Autodesk Fusion 360 part; units mm, degrees
note: some values were not read from the file. Chosen so that the rebuilt part matches the saved one: which bodies a step acts on; a direction. Set by a fixed rule: which sketch regions a step uses.
(part 2 of 5)
sketch "ToF block FL sketch" plane through (0, 0, 0) normal (0, 0, 1) x (1, 0, 0) in component "Upper frame"
  line L0 (88.4256, 25.8962) -> (99.9126, 31.2979)
  line L1 (99.9126, 31.2979) -> (89.9042, 53.4861)
  line L2 (89.9042, 53.4861) -> (78.1222, 47.992)
  line L3 (78.1222, 47.992) -> (88.4256, 25.8962)
extrude "ToF block FL" add sketch "ToF block FL sketch" along normal blind 30 from surface at 87 bodies 44 in component "Upper frame"
sketch "ToF block FR sketch" plane through (0, 0, 0) normal (0, 0, 1) x (1, 0, 0) in component "Upper frame"
  line L0 (78.1222, -47.992) -> (89.9042, -53.4861)
  line L1 (89.9042, -53.4861) -> (99.9126, -31.2979)
  line L2 (99.9126, -31.2979) -> (88.4256, -25.8962)
  line L3 (88.4256, -25.8962) -> (78.1222, -47.992)
extrude "ToF block FR" add sketch "ToF block FR sketch" along normal blind 30 from surface at 87 bodies 44 in component "Upper frame"
sketch "ToF block SFL sketch" plane through (0, 0, 0) normal (0, 0, 1) x (1, 0, 0) in component "Upper frame"
  line L0 (80.69, 53.1) -> (80.69, 66.1)
  line L1 (80.69, 66.1) -> (56.31, 66.1)
  line L2 (56.31, 66.1) -> (56.31, 53.1)
  line L3 (56.31, 53.1) -> (80.69, 53.1)
extrude "ToF block SFL" add sketch "ToF block SFL sketch" along normal blind 30 from surface at 87 bodies 44 in component "Upper frame"
sketch "ToF block SFR sketch" plane through (0, 0, 0) normal (0, 0, 1) x (1, 0, 0) in component "Upper frame"
  line L0 (56.31, -53.1) -> (56.31, -66.1)
  line L1 (56.31, -66.1) -> (80.69, -66.1)
  line L2 (80.69, -66.1) -> (80.69, -53.1)
  line L3 (80.69, -53.1) -> (56.31, -53.1)
extrude "ToF block SFR" add sketch "ToF block SFR sketch" along normal blind 30 from surface at 87 bodies 44 in component "Upper frame"
sketch "ToF block SRL sketch" plane through (0, 0, 0) normal (0, 0, 1) x (1, 0, 0) in component "Upper frame"
  line L0 (-56.31, 53.1) -> (-56.31, 66.1)
  line L1 (-56.31, 66.1) -> (-80.69, 66.1)
  line L2 (-80.69, 66.1) -> (-80.69, 53.1)
  line L3 (-80.69, 53.1) -> (-56.31, 53.1)
extrude "ToF block SRL" add sketch "ToF block SRL sketch" along normal blind 30 from surface at 87 bodies 44 in component "Upper frame"
sketch "ToF block SRR sketch" plane through (0, 0, 0) normal (0, 0, 1) x (1, 0, 0) in component "Upper frame"
  line L0 (-80.69, -53.1) -> (-80.69, -66.1)
  line L1 (-80.69, -66.1) -> (-56.31, -66.1)
  line L2 (-56.31, -66.1) -> (-56.31, -53.1)
  line L3 (-56.31, -53.1) -> (-80.69, -53.1)
extrude "ToF block SRR" add sketch "ToF block SRR sketch" along normal blind 30 from surface at 87 bodies 44 in component "Upper frame"
sketch "ToF block RL sketch" plane through (0, 0, 0) normal (0, 0, 1) x (1, 0, 0) in component "Upper frame"
  line L0 (-77.1, 48.19) -> (-90.1, 48.19)
  line L1 (-90.1, 48.19) -> (-90.1, 23.81)
  line L2 (-90.1, 23.81) -> (-77.1, 23.81)
  line L3 (-77.1, 23.81) -> (-77.1, 48.19)
extrude "ToF block RL" add sketch "ToF block RL sketch" along normal blind 30 from surface at 87 bodies 44 in component "Upper frame"
sketch "ToF block RR sketch" plane through (0, 0, 0) normal (0, 0, 1) x (1, 0, 0) in component "Upper frame"
  line L0 (-77.1, -23.81) -> (-90.1, -23.81)
  line L1 (-90.1, -23.81) -> (-90.1, -48.19)
  line L2 (-90.1, -48.19) -> (-77.1, -48.19)
  line L3 (-77.1, -48.19) -> (-77.1, -23.81)
extrude "ToF block RR" add sketch "ToF block RR sketch" along normal blind 30 from surface at 87 bodies 44 in component "Upper frame"
sketch "Seat rebate 0 sketch" plane through (0, 0, 0) normal (0, 0, 1) x (1, 0, 0) in component "Upper frame"
  line L0 (31.5, 8) -> (39.5, 8)
  line L1 (39.5, 8) -> (39.5, 13)
  line L2 (39.5, 13) -> (31.5, 13)
  line L3 (31.5, 13) -> (31.5, 8)
extrude "Seat rebate 0" cut sketch "Seat rebate 0 sketch" along normal blind 2.5 from surface at 88.5 bodies 44 in component "Upper frame"
sketch "Seat rebate 1 sketch" plane through (0, 0, 0) normal (0, 0, 1) x (1, 0, 0) in component "Upper frame"
  line L0 (31.5, -13) -> (39.5, -13)
  line L1 (39.5, -13) -> (39.5, -8)
  line L2 (39.5, -8) -> (31.5, -8)
  line L3 (31.5, -8) -> (31.5, -13)
extrude "Seat rebate 1" cut sketch "Seat rebate 1 sketch" along normal blind 2.5 from surface at 88.5 bodies 44 in component "Upper frame"
sketch "Seat rebate 2 sketch" plane through (0, 0, 0) normal (0, 0, 1) x (1, 0, 0) in component "Upper frame"
  line L0 (-75.5, -5.5) -> (-71.5, -5.5)
  line L1 (-71.5, -5.5) -> (-71.5, 5.5)
  line L2 (-71.5, 5.5) -> (-75.5, 5.5)
  line L3 (-75.5, 5.5) -> (-75.5, -5.5)
extrude "Seat rebate 2" cut sketch "Seat rebate 2 sketch" along normal blind 2.5 from surface at 88.5 bodies 44 in component "Upper frame"
sketch "Screw hole +12 sketch" plane through (0, 0, 0) normal (0, 0, 1) x (1, 0, 0) in component "Upper frame"
  circle A0 centre (95.3694, 20.2714) radius 1.65
extrude "Screw hole +12" cut sketch "Screw hole +12 sketch" along normal blind 32 from surface at 86 bodies 44 in component "Upper frame"
sketch "Screw counterbore +12 sketch" plane through (0, 0, 0) normal (0, 0, 1) x (1, 0, 0) in component "Upper frame"
  circle A0 centre (95.3694, 20.2714) radius 3
extrude "Screw counterbore +12" cut sketch "Screw counterbore +12 sketch" along normal blind 4 from surface at 114 bodies 44 in component "Upper frame"
sketch "Screw hole +60 sketch" plane through (0, 0, 0) normal (0, 0, 1) x (1, 0, 0) in component "Upper frame"
  circle A0 centre (48.75, 84.4375) radius 1.65
extrude "Screw hole +60" cut sketch "Screw hole +60 sketch" along normal blind 32 from surface at 86 bodies 44 in component "Upper frame"
sketch "Screw counterbore +60 sketch" plane through (0, 0, 0) normal (0, 0, 1) x (1, 0, 0) in component "Upper frame"
  circle A0 centre (48.75, 84.4375) radius 3
extrude "Screw counterbore +60" cut sketch "Screw counterbore +60 sketch" along normal blind 4 from surface at 114 bodies 44 in component "Upper frame"
sketch "Screw hole +118 sketch" plane through (0, 0, 0) normal (0, 0, 1) x (1, 0, 0) in component "Upper frame"
  circle A0 centre (-45.7735, 86.0874) radius 1.65
extrude "Screw hole +118" cut sketch "Screw hole +118 sketch" along normal blind 32 from surface at 86 bodies 44 in component "Upper frame"
sketch "Screw counterbore +118 sketch" plane through (0, 0, 0) normal (0, 0, 1) x (1, 0, 0) in component "Upper frame"
  circle A0 centre (-45.7735, 86.0874) radius 3
extrude "Screw counterbore +118" cut sketch "Screw counterbore +118 sketch" along normal blind 4 from surface at 114 bodies 44 in component "Upper frame"
sketch "Screw hole -12 sketch" plane through (0, 0, 0) normal (0, 0, 1) x (1, 0, 0) in component "Upper frame"
  circle A0 centre (95.3694, -20.2714) radius 1.65
extrude "Screw hole -12" cut sketch "Screw hole -12 sketch" along normal blind 32 from surface at 86 bodies 44 in component "Upper frame"
sketch "Screw counterbore -12 sketch" plane through (0, 0, 0) normal (0, 0, 1) x (1, 0, 0) in component "Upper frame"
  circle A0 centre (95.3694, -20.2714) radius 3
extrude "Screw counterbore -12" cut sketch "Screw counterbore -12 sketch" along normal blind 4 from surface at 114 bodies 44 in component "Upper frame"
sketch "Screw hole -60 sketch" plane through (0, 0, 0) normal (0, 0, 1) x (1, 0, 0) in component "Upper frame"
  circle A0 centre (48.75, -84.4375) radius 1.65
extrude "Screw hole -60" cut sketch "Screw hole -60 sketch" along normal blind 32 from surface at 86 bodies 44 in component "Upper frame"
sketch "Screw counterbore -60 sketch" plane through (0, 0, 0) normal (0, 0, 1) x (1, 0, 0) in component "Upper frame"
  circle A0 centre (48.75, -84.4375) radius 3
extrude "Screw counterbore -60" cut sketch "Screw counterbore -60 sketch" along normal blind 4 from surface at 114 bodies 44 in component "Upper frame"
sketch "Screw hole -118 sketch" plane through (0, 0, 0) normal (0, 0, 1) x (1, 0, 0) in component "Upper frame"
  circle A0 centre (-45.7735, -86.0874) radius 1.65
extrude "Screw hole -118" cut sketch "Screw hole -118 sketch" along normal blind 32 from surface at 86 bodies 44 in component "Upper frame"
sketch "Screw counterbore -118 sketch" plane through (0, 0, 0) normal (0, 0, 1) x (1, 0, 0) in component "Upper frame"
  circle A0 centre (-45.7735, -86.0874) radius 3
extrude "Screw counterbore -118" cut sketch "Screw counterbore -118 sketch" along normal blind 4 from surface at 114 bodies 44 in component "Upper frame"
sketch "Hook rebate +71 sketch" plane through (0, 0, 0) normal (0, 0, 1) x (1, 0, 0) in component "Upper frame"
  arc A0 (44.7975, 96.0686) -> (23.8448, 103.2832) centre (0, 0) ccw
  line L0 (23.8448, 103.2832) -> (23.2599, 100.7499)
  arc A1 (43.6987, 93.7122) -> (23.2599, 100.7499) centre (0, 0) ccw
  line L1 (43.6987, 93.7122) -> (44.7975, 96.0686)
extrude "Hook rebate +71" cut sketch "Hook rebate +71 sketch" along normal blind 9 from surface at 109 bodies 44 in component "Upper frame"
sketch "Hook groove +71 sketch" plane through (0, 0, 0) normal (0, 0, 1) x (1, 0, 0) in component "Upper frame"
  arc A0 (41.2705, 94.9157) -> (25.9143, 100.2033) centre (0, 0) ccw
  line L0 (25.9143, 100.2033) -> (25.6389, 99.1383)
  arc A1 (40.8319, 93.907) -> (25.6389, 99.1383) centre (0, 0) ccw
  line L1 (40.8319, 93.907) -> (41.2705, 94.9157)
extrude "Hook groove +71" cut sketch "Hook groove +71 sketch" along normal blind 3 from surface at 110.5 bodies 44 in component "Upper frame"
sketch "Hook rebate +114 sketch" plane through (0, 0, 0) normal (0, 0, 1) x (1, 0, 0) in component "Upper frame"
  arc A0 (-32.7558, 100.812) -> (-53, 91.7987) centre (0, 0) ccw
  line L0 (-53, 91.7987) -> (-51.7, 89.547)
  arc A1 (-31.9524, 98.3392) -> (-51.7, 89.547) centre (0, 0) ccw
  line L1 (-31.9524, 98.3392) -> (-32.7558, 100.812)
extrude "Hook rebate +114" cut sketch "Hook rebate +114 sketch" along normal blind 9 from surface at 109 bodies 44 in component "Upper frame"
sketch "Hook groove +114 sketch" plane through (0, 0, 0) normal (0, 0, 1) x (1, 0, 0) in component "Upper frame"
  arc A0 (-34.549, 97.5634) -> (-49.3859, 90.9576) centre (0, 0) ccw
  line L0 (-49.3859, 90.9576) -> (-48.8611, 89.9909)
  arc A1 (-34.1818, 96.5265) -> (-48.8611, 89.9909) centre (0, 0) ccw
  line L1 (-34.1818, 96.5265) -> (-34.549, 97.5634)
extrude "Hook groove +114" cut sketch "Hook groove +114 sketch" along normal blind 3 from surface at 110.5 bodies 44 in component "Upper frame"
sketch "Hook rebate -71 sketch" plane through (0, 0, 0) normal (0, 0, 1) x (1, 0, 0) in component "Upper frame"
  arc A0 (23.8448, -103.2832) -> (44.7975, -96.0686) centre (0, 0) ccw
  line L0 (44.7975, -96.0686) -> (43.6987, -93.7122)
  arc A1 (23.2599, -100.7499) -> (43.6987, -93.7122) centre (0, 0) ccw
  line L1 (23.2599, -100.7499) -> (23.8448, -103.2832)
extrude "Hook rebate -71" cut sketch "Hook rebate -71 sketch" along normal blind 9 from surface at 109 bodies 44 in component "Upper frame"
sketch "Hook groove -71 sketch" plane through (0, 0, 0) normal (0, 0, 1) x (1, 0, 0) in component "Upper frame"
  arc A0 (25.9143, -100.2033) -> (41.2705, -94.9157) centre (0, 0) ccw
  line L0 (41.2705, -94.9157) -> (40.8319, -93.907)
  arc A1 (25.6389, -99.1383) -> (40.8319, -93.907) centre (0, 0) ccw
  line L1 (25.6389, -99.1383) -> (25.9143, -100.2033)
extrude "Hook groove -71" cut sketch "Hook groove -71 sketch" along normal blind 3 from surface at 110.5 bodies 44 in component "Upper frame"
sketch "Hook rebate -114 sketch" plane through (0, 0, 0) normal (0, 0, 1) x (1, 0, 0) in component "Upper frame"
  arc A0 (-53, -91.7987) -> (-32.7558, -100.812) centre (0, 0) ccw
  line L0 (-32.7558, -100.812) -> (-31.9524, -98.3392)
  arc A1 (-51.7, -89.547) -> (-31.9524, -98.3392) centre (0, 0) ccw
  line L1 (-51.7, -89.547) -> (-53, -91.7987)
extrude "Hook rebate -114" cut sketch "Hook rebate -114 sketch" along normal blind 9 from surface at 109 bodies 44 in component "Upper frame"
sketch "Hook groove -114 sketch" plane through (0, 0, 0) normal (0, 0, 1) x (1, 0, 0) in component "Upper frame"
  arc A0 (-49.3859, -90.9576) -> (-34.549, -97.5634) centre (0, 0) ccw
  line L0 (-34.549, -97.5634) -> (-34.1818, -96.5265)
  arc A1 (-48.8611, -89.9909) -> (-34.1818, -96.5265) centre (0, 0) ccw
  line L1 (-48.8611, -89.9909) -> (-49.3859, -90.9576)
extrude "Hook groove -114" cut sketch "Hook groove -114 sketch" along normal blind 3 from surface at 110.5 bodies 44 in component "Upper frame"
sketch "ToF pocket F sketch" plane through (0, 0, 0) normal (0, 0, 1) x (1, 0, 0) in component "Upper frame"
  line L0 (91.1, -9.69) -> (98.6, -9.69)
  line L1 (98.6, -9.69) -> (98.6, 9.69)
  line L2 (98.6, 9.69) -> (91.1, 9.69)
  line L3 (91.1, 9.69) -> (91.1, -9.69)
extrude "ToF pocket F" cut sketch "ToF pocket F sketch" along normal blind 28 from surface at 90 bodies 44 in component "Upper frame"
sketch "ToF plug shaft F sketch" plane through (0, 0, 0) normal (0, 0, 1) x (1, 0, 0) in component "Upper frame"
  line L0 (94.5, -3.8) -> (99, -3.8)
  line L1 (99, -3.8) -> (99, 3.8)
  line L2 (99, 3.8) -> (94.5, 3.8)
  line L3 (94.5, 3.8) -> (94.5, -3.8)
extrude "ToF plug shaft F" cut sketch "ToF plug shaft F sketch" along normal blind 4.5 from surface at 86 bodies 44 in component "Upper frame"
sketch "ToF tunnel F sketch" plane through (0, 0, 0) normal (0, 0, 1) x (1, 0, 0) in component "Upper frame"
  line L0 (98.1, -9) -> (135, -9)
  line L1 (135, -9) -> (135, 9)
  line L2 (135, 9) -> (98.1, 9)
  line L3 (98.1, 9) -> (98.1, -9)
extrude "ToF tunnel F" cut sketch "ToF tunnel F sketch" along normal blind 18 from surface at 93.8 bodies 44 in component "Upper frame"
sketch "ToF posts F sketch" plane through (0, 0, 0) normal (0, 0, 1) x (1, 0, 0) in component "Upper frame"
  line L0 (95, 3.75) -> (99.2, 3.75)
  line L1 (99.2, 3.75) -> (99.2, 8.95)
  line L2 (99.2, 8.95) -> (95, 8.95)
  line L3 (95, 8.95) -> (95, 3.75)
  line L4 (95, -8.95) -> (99.2, -8.95)
  line L5 (99.2, -8.95) -> (99.2, -3.75)
  line L6 (99.2, -3.75) -> (95, -3.75)
  line L7 (95, -3.75) -> (95, -8.95)
extrude "ToF posts F" add sketch "ToF posts F sketch" along normal blind 5.2 from surface at 110.36 bodies 44 in component "Upper frame"
sketch "ToF pilots F sketch" plane through (0, 0, 0) normal (0, 0, 1) x (1, 0, 0) in component "Upper frame"
  line L0 (94.5, 5.25) -> (99.5, 5.25)
  line L1 (99.5, 5.25) -> (99.5, 7.45)
  line L2 (99.5, 7.45) -> (94.5, 7.45)
  line L3 (94.5, 7.45) -> (94.5, 5.25)
  line L4 (94.5, -7.45) -> (99.5, -7.45)
  line L5 (99.5, -7.45) -> (99.5, -5.25)
  line L6 (99.5, -5.25) -> (94.5, -5.25)
  line L7 (94.5, -5.25) -> (94.5, -7.45)
extrude "ToF pilots F" cut sketch "ToF pilots F sketch" along normal blind 2.2 from surface at 111.86 bodies 44 in component "Upper frame"
sketch "ToF screw access F sketch" plane through (0, 0, 0) normal (0, 0, 1) x (1, 0, 0) in component "Upper frame"
  line L0 (87.6, 3.85) -> (91.3, 3.85)
  line L1 (91.3, 3.85) -> (91.3, 8.85)
  line L2 (91.3, 8.85) -> (87.6, 8.85)
  line L3 (87.6, 8.85) -> (87.6, 3.85)
  line L4 (87.6, -8.85) -> (91.3, -8.85)
  line L5 (91.3, -8.85) -> (91.3, -3.85)
  line L6 (91.3, -3.85) -> (87.6, -3.85)
  line L7 (87.6, -3.85) -> (87.6, -8.85)
extrude "ToF screw access F" cut sketch "ToF screw access F sketch" along normal blind 5 from surface at 110.46 bodies 44 in component "Upper frame"
sketch "ToF pocket FL sketch" plane through (0, 0, 0) normal (0, 0, 1) x (1, 0, 0) in component "Upper frame"
  line L0 (90.088, 29.4299) -> (96.8853, 32.5995)
  line L1 (96.8853, 32.5995) -> (88.695, 50.1637)
  line L2 (88.695, 50.1637) -> (81.8977, 46.9941)
  line L3 (81.8977, 46.9941) -> (90.088, 29.4299)
extrude "ToF pocket FL" cut sketch "ToF pocket FL sketch" along normal blind 28 from surface at 90 bodies 44 in component "Upper frame"
sketch "ToF plug shaft FL sketch" plane through (0, 0, 0) normal (0, 0, 1) x (1, 0, 0) in component "Upper frame"
  line L0 (90.6803, 36.2049) -> (94.7586, 38.1067)
  line L1 (94.7586, 38.1067) -> (91.5467, 44.9946)
  line L2 (91.5467, 44.9946) -> (87.4684, 43.0929)
  line L3 (87.4684, 43.0929) -> (90.6803, 36.2049)
extrude "ToF plug shaft FL" cut sketch "ToF plug shaft FL sketch" along normal blind 4.5 from surface at 86 bodies 44 in component "Upper frame"
sketch "ToF tunnel FL sketch" plane through (0, 0, 0) normal (0, 0, 1) x (1, 0, 0) in component "Upper frame"
  line L0 (96.1406, 33.0135) -> (129.5833, 48.6082)
  line L1 (129.5833, 48.6082) -> (121.9762, 64.9217)
  line L2 (121.9762, 64.9217) -> (88.5334, 49.3271)
  line L3 (88.5334, 49.3271) -> (96.1406, 33.0135)
extrude "ToF tunnel FL" cut sketch "ToF tunnel FL sketch" along normal blind 18 from surface at 93.8 bodies 44 in component "Upper frame"
sketch "ToF posts FL sketch" plane through (0, 0, 0) normal (0, 0, 1) x (1, 0, 0) in component "Upper frame"
  line L0 (87.9426, 43.2588) -> (91.7491, 45.0338)
  line L1 (91.7491, 45.0338) -> (89.5515, 49.7466)
  line L2 (89.5515, 49.7466) -> (85.745, 47.9716)
  line L3 (85.745, 47.9716) -> (87.9426, 43.2588)
  line L4 (93.3099, 31.7487) -> (97.1164, 33.5237)
  line L5 (97.1164, 33.5237) -> (94.9188, 38.2365)
  line L6 (94.9188, 38.2365) -> (91.1123, 36.4615)
  line L7 (91.1123, 36.4615) -> (93.3099, 31.7487)
extrude "ToF posts FL" add sketch "ToF posts FL sketch" along normal blind 5.2 from surface at 110.36 bodies 44 in component "Upper frame"
sketch "ToF pilots FL sketch" plane through (0, 0, 0) normal (0, 0, 1) x (1, 0, 0) in component "Upper frame"
  line L0 (86.8556, 44.407) -> (91.3871, 46.5201)
  line L1 (91.3871, 46.5201) -> (90.4573, 48.514)
  line L2 (90.4573, 48.514) -> (85.9258, 46.4009)
  line L3 (85.9258, 46.4009) -> (86.8556, 44.407)
  line L4 (92.2228, 32.8969) -> (96.7543, 35.01)
  line L5 (96.7543, 35.01) -> (95.8246, 37.0039)
  line L6 (95.8246, 37.0039) -> (91.293, 34.8908)
  line L7 (91.293, 34.8908) -> (92.2228, 32.8969)
extrude "ToF pilots FL" cut sketch "ToF pilots FL sketch" along normal blind 2.2 from surface at 111.86 bodies 44 in component "Upper frame"
sketch "ToF screw access FL sketch" plane through (0, 0, 0) normal (0, 0, 1) x (1, 0, 0) in component "Upper frame"
  line L0 (81.1937, 40.2221) -> (84.547, 41.7858)
  line L1 (84.547, 41.7858) -> (82.4339, 46.3173)
  line L2 (82.4339, 46.3173) -> (79.0806, 44.7536)
  line L3 (79.0806, 44.7536) -> (81.1937, 40.2221)
  line L4 (86.5609, 28.712) -> (89.9143, 30.2757)
  line L5 (89.9143, 30.2757) -> (87.8012, 34.8072)
  line L6 (87.8012, 34.8072) -> (84.4479, 33.2435)
  line L7 (84.4479, 33.2435) -> (86.5609, 28.712)
extrude "ToF screw access FL" cut sketch "ToF screw access FL sketch" along normal blind 5 from surface at 110.46 bodies 44 in component "Upper frame"
sketch "ToF pocket FR sketch" plane through (0, 0, 0) normal (0, 0, 1) x (1, 0, 0) in component "Upper frame"
  line L0 (81.8977, -46.9941) -> (88.695, -50.1637)
  line L1 (88.695, -50.1637) -> (96.8853, -32.5995)
  line L2 (96.8853, -32.5995) -> (90.088, -29.4299)
  line L3 (90.088, -29.4299) -> (81.8977, -46.9941)
extrude "ToF pocket FR" cut sketch "ToF pocket FR sketch" along normal blind 28 from surface at 90 bodies 44 in component "Upper frame"
sketch "ToF plug shaft FR sketch" plane through (0, 0, 0) normal (0, 0, 1) x (1, 0, 0) in component "Upper frame"
  line L0 (87.4684, -43.0929) -> (91.5467, -44.9946)
  line L1 (91.5467, -44.9946) -> (94.7586, -38.1067)
  line L2 (94.7586, -38.1067) -> (90.6803, -36.2049)
  line L3 (90.6803, -36.2049) -> (87.4684, -43.0929)
extrude "ToF plug shaft FR" cut sketch "ToF plug shaft FR sketch" along normal blind 4.5 from surface at 86 bodies 44 in component "Upper frame"
sketch "ToF tunnel FR sketch" plane through (0, 0, 0) normal (0, 0, 1) x (1, 0, 0) in component "Upper frame"
  line L0 (88.5334, -49.3271) -> (121.9762, -64.9217)
  line L1 (121.9762, -64.9217) -> (129.5833, -48.6082)
  line L2 (129.5833, -48.6082) -> (96.1406, -33.0135)
  line L3 (96.1406, -33.0135) -> (88.5334, -49.3271)
extrude "ToF tunnel FR" cut sketch "ToF tunnel FR sketch" along normal blind 18 from surface at 93.8 bodies 44 in component "Upper frame"
sketch "ToF posts FR sketch" plane through (0, 0, 0) normal (0, 0, 1) x (1, 0, 0) in component "Upper frame"
  line L0 (91.1123, -36.4615) -> (94.9188, -38.2365)
  line L1 (94.9188, -38.2365) -> (97.1164, -33.5237)
  line L2 (97.1164, -33.5237) -> (93.3099, -31.7487)
  line L3 (93.3099, -31.7487) -> (91.1123, -36.4615)
  line L4 (85.745, -47.9716) -> (89.5515, -49.7466)
  line L5 (89.5515, -49.7466) -> (91.7491, -45.0338)
  line L6 (91.7491, -45.0338) -> (87.9426, -43.2588)
  line L7 (87.9426, -43.2588) -> (85.745, -47.9716)
extrude "ToF posts FR" add sketch "ToF posts FR sketch" along normal blind 5.2 from surface at 110.36 bodies 44 in component "Upper frame"
sketch "ToF pilots FR sketch" plane through (0, 0, 0) normal (0, 0, 1) x (1, 0, 0) in component "Upper frame"
  line L0 (91.293, -34.8908) -> (95.8246, -37.0039)
  line L1 (95.8246, -37.0039) -> (96.7543, -35.01)
  line L2 (96.7543, -35.01) -> (92.2228, -32.8969)
  line L3 (92.2228, -32.8969) -> (91.293, -34.8908)
  line L4 (85.9258, -46.4009) -> (90.4573, -48.514)
  line L5 (90.4573, -48.514) -> (91.3871, -46.5201)
  line L6 (91.3871, -46.5201) -> (86.8556, -44.407)
  line L7 (86.8556, -44.407) -> (85.9258, -46.4009)
extrude "ToF pilots FR" cut sketch "ToF pilots FR sketch" along normal blind 2.2 from surface at 111.86 bodies 44 in component "Upper frame"
sketch "ToF screw access FR sketch" plane through (0, 0, 0) normal (0, 0, 1) x (1, 0, 0) in component "Upper frame"
  line L0 (84.4479, -33.2435) -> (87.8012, -34.8072)
  line L1 (87.8012, -34.8072) -> (89.9143, -30.2757)
  line L2 (89.9143, -30.2757) -> (86.5609, -28.712)
  line L3 (86.5609, -28.712) -> (84.4479, -33.2435)
  line L4 (79.0806, -44.7536) -> (82.4339, -46.3173)
  line L5 (82.4339, -46.3173) -> (84.547, -41.7858)
  line L6 (84.547, -41.7858) -> (81.1937, -40.2221)
  line L7 (81.1937, -40.2221) -> (79.0806, -44.7536)
extrude "ToF screw access FR" cut sketch "ToF screw access FR sketch" along normal blind 5 from surface at 110.46 bodies 44 in component "Upper frame"
sketch "ToF pocket SFL sketch" plane through (0, 0, 0) normal (0, 0, 1) x (1, 0, 0) in component "Upper frame"
  line L0 (78.19, 56.1) -> (78.19, 63.6)
  line L1 (78.19, 63.6) -> (58.81, 63.6)
  line L2 (58.81, 63.6) -> (58.81, 56.1)
  line L3 (58.81, 56.1) -> (78.19, 56.1)
extrude "ToF pocket SFL" cut sketch "ToF pocket SFL sketch" along normal blind 28 from surface at 90 bodies 44 in component "Upper frame"
sketch "ToF plug shaft SFL sketch" plane through (0, 0, 0) normal (0, 0, 1) x (1, 0, 0) in component "Upper frame"
  line L0 (72.3, 59.5) -> (72.3, 64)
  line L1 (72.3, 64) -> (64.7, 64)
  line L2 (64.7, 64) -> (64.7, 59.5)
  line L3 (64.7, 59.5) -> (72.3, 59.5)
extrude "ToF plug shaft SFL" cut sketch "ToF plug shaft SFL sketch" along normal blind 4.5 from surface at 86 bodies 44 in component "Upper frame"
sketch "ToF tunnel SFL sketch" plane through (0, 0, 0) normal (0, 0, 1) x (1, 0, 0) in component "Upper frame"
  line L0 (77.5, 63.1) -> (77.5, 100)
  line L1 (77.5, 100) -> (59.5, 100)
  line L2 (59.5, 100) -> (59.5, 63.1)
  line L3 (59.5, 63.1) -> (77.5, 63.1)
extrude "ToF tunnel SFL" cut sketch "ToF tunnel SFL sketch" along normal blind 18 from surface at 93.8 bodies 44 in component "Upper frame"
sketch "ToF posts SFL sketch" plane through (0, 0, 0) normal (0, 0, 1) x (1, 0, 0) in component "Upper frame"
  line L0 (64.75, 60) -> (64.75, 64.2)
  line L1 (64.75, 64.2) -> (59.55, 64.2)
  line L2 (59.55, 64.2) -> (59.55, 60)
  line L3 (59.55, 60) -> (64.75, 60)
  line L4 (77.45, 60) -> (77.45, 64.2)
  line L5 (77.45, 64.2) -> (72.25, 64.2)
  line L6 (72.25, 64.2) -> (72.25, 60)
  line L7 (72.25, 60) -> (77.45, 60)
extrude "ToF posts SFL" add sketch "ToF posts SFL sketch" along normal blind 5.2 from surface at 110.36 bodies 44 in component "Upper frame"
sketch "ToF pilots SFL sketch" plane through (0, 0, 0) normal (0, 0, 1) x (1, 0, 0) in component "Upper frame"
  line L0 (63.25, 59.5) -> (63.25, 64.5)
  line L1 (63.25, 64.5) -> (61.05, 64.5)
  line L2 (61.05, 64.5) -> (61.05, 59.5)
  line L3 (61.05, 59.5) -> (63.25, 59.5)
  line L4 (75.95, 59.5) -> (75.95, 64.5)
  line L5 (75.95, 64.5) -> (73.75, 64.5)
  line L6 (73.75, 64.5) -> (73.75, 59.5)
  line L7 (73.75, 59.5) -> (75.95, 59.5)
extrude "ToF pilots SFL" cut sketch "ToF pilots SFL sketch" along normal blind 2.2 from surface at 111.86 bodies 44 in component "Upper frame"
sketch "ToF screw access SFL sketch" plane through (0, 0, 0) normal (0, 0, 1) x (1, 0, 0) in component "Upper frame"
  line L0 (64.65, 52.6) -> (64.65, 56.3)
  line L1 (64.65, 56.3) -> (59.65, 56.3)
  line L2 (59.65, 56.3) -> (59.65, 52.6)
  line L3 (59.65, 52.6) -> (64.65, 52.6)
  line L4 (77.35, 52.6) -> (77.35, 56.3)
  line L5 (77.35, 56.3) -> (72.35, 56.3)
  line L6 (72.35, 56.3) -> (72.35, 52.6)
  line L7 (72.35, 52.6) -> (77.35, 52.6)
extrude "ToF screw access SFL" cut sketch "ToF screw access SFL sketch" along normal blind 5 from surface at 110.46 bodies 44 in component "Upper frame"
sketch "ToF pocket SFR sketch" plane through (0, 0, 0) normal (0, 0, 1) x (1, 0, 0) in component "Upper frame"
  line L0 (58.81, -56.1) -> (58.81, -63.6)
  line L1 (58.81, -63.6) -> (78.19, -63.6)
  line L2 (78.19, -63.6) -> (78.19, -56.1)
  line L3 (78.19, -56.1) -> (58.81, -56.1)
extrude "ToF pocket SFR" cut sketch "ToF pocket SFR sketch" along normal blind 28 from surface at 90 bodies 44 in component "Upper frame"
sketch "ToF plug shaft SFR sketch" plane through (0, 0, 0) normal (0, 0, 1) x (1, 0, 0) in component "Upper frame"
  line L0 (64.7, -59.5) -> (64.7, -64)
  line L1 (64.7, -64) -> (72.3, -64)
  line L2 (72.3, -64) -> (72.3, -59.5)
  line L3 (72.3, -59.5) -> (64.7, -59.5)
extrude "ToF plug shaft SFR" cut sketch "ToF plug shaft SFR sketch" along normal blind 4.5 from surface at 86 bodies 44 in component "Upper frame"
sketch "ToF tunnel SFR sketch" plane through (0, 0, 0) normal (0, 0, 1) x (1, 0, 0) in component "Upper frame"
  line L0 (59.5, -63.1) -> (59.5, -100)
  line L1 (59.5, -100) -> (77.5, -100)
  line L2 (77.5, -100) -> (77.5, -63.1)
  line L3 (77.5, -63.1) -> (59.5, -63.1)
extrude "ToF tunnel SFR" cut sketch "ToF tunnel SFR sketch" along normal blind 18 from surface at 93.8 bodies 44 in component "Upper frame"
sketch "ToF posts SFR sketch" plane through (0, 0, 0) normal (0, 0, 1) x (1, 0, 0) in component "Upper frame"
  line L0 (72.25, -60) -> (72.25, -64.2)
  line L1 (72.25, -64.2) -> (77.45, -64.2)
  line L2 (77.45, -64.2) -> (77.45, -60)
  line L3 (77.45, -60) -> (72.25, -60)
  line L4 (59.55, -60) -> (59.55, -64.2)
  line L5 (59.55, -64.2) -> (64.75, -64.2)
  line L6 (64.75, -64.2) -> (64.75, -60)
  line L7 (64.75, -60) -> (59.55, -60)
extrude "ToF posts SFR" add sketch "ToF posts SFR sketch" along normal blind 5.2 from surface at 110.36 bodies 44 in component "Upper frame"
sketch "ToF pilots SFR sketch" plane through (0, 0, 0) normal (0, 0, 1) x (1, 0, 0) in component "Upper frame"
  line L0 (73.75, -59.5) -> (73.75, -64.5)
  line L1 (73.75, -64.5) -> (75.95, -64.5)
  line L2 (75.95, -64.5) -> (75.95, -59.5)
  line L3 (75.95, -59.5) -> (73.75, -59.5)
  line L4 (61.05, -59.5) -> (61.05, -64.5)
  line L5 (61.05, -64.5) -> (63.25, -64.5)
  line L6 (63.25, -64.5) -> (63.25, -59.5)
  line L7 (63.25, -59.5) -> (61.05, -59.5)
extrude "ToF pilots SFR" cut sketch "ToF pilots SFR sketch" along normal blind 2.2 from surface at 111.86 bodies 44 in component "Upper frame"
sketch "ToF screw access SFR sketch" plane through (0, 0, 0) normal (0, 0, 1) x (1, 0, 0) in component "Upper frame"
  line L0 (72.35, -52.6) -> (72.35, -56.3)
  line L1 (72.35, -56.3) -> (77.35, -56.3)
  line L2 (77.35, -56.3) -> (77.35, -52.6)
  line L3 (77.35, -52.6) -> (72.35, -52.6)
  line L4 (59.65, -52.6) -> (59.65, -56.3)
  line L5 (59.65, -56.3) -> (64.65, -56.3)
  line L6 (64.65, -56.3) -> (64.65, -52.6)
  line L7 (64.65, -52.6) -> (59.65, -52.6)
extrude "ToF screw access SFR" cut sketch "ToF screw access SFR sketch" along normal blind 5 from surface at 110.46 bodies 44 in component "Upper frame"
sketch "ToF pocket SRL sketch" plane through (0, 0, 0) normal (0, 0, 1) x (1, 0, 0) in component "Upper frame"
  line L0 (-58.81, 56.1) -> (-58.81, 63.6)
  line L1 (-58.81, 63.6) -> (-78.19, 63.6)
  line L2 (-78.19, 63.6) -> (-78.19, 56.1)
  line L3 (-78.19, 56.1) -> (-58.81, 56.1)
extrude "ToF pocket SRL" cut sketch "ToF pocket SRL sketch" along normal blind 28 from surface at 90 bodies 44 in component "Upper frame"
sketch "ToF plug shaft SRL sketch" plane through (0, 0, 0) normal (0, 0, 1) x (1, 0, 0) in component "Upper frame"
  line L0 (-64.7, 59.5) -> (-64.7, 64)
  line L1 (-64.7, 64) -> (-72.3, 64)
  line L2 (-72.3, 64) -> (-72.3, 59.5)
  line L3 (-72.3, 59.5) -> (-64.7, 59.5)
extrude "ToF plug shaft SRL" cut sketch "ToF plug shaft SRL sketch" along normal blind 4.5 from surface at 86 bodies 44 in component "Upper frame"
sketch "ToF tunnel SRL sketch" plane through (0, 0, 0) normal (0, 0, 1) x (1, 0, 0) in component "Upper frame"
  line L0 (-59.5, 63.1) -> (-59.5, 100)
  line L1 (-59.5, 100) -> (-77.5, 100)
  line L2 (-77.5, 100) -> (-77.5, 63.1)
  line L3 (-77.5, 63.1) -> (-59.5, 63.1)
extrude "ToF tunnel SRL" cut sketch "ToF tunnel SRL sketch" along normal blind 18 from surface at 93.8 bodies 44 in component "Upper frame"
sketch "ToF posts SRL sketch" plane through (0, 0, 0) normal (0, 0, 1) x (1, 0, 0) in component "Upper frame"
  line L0 (-72.25, 60) -> (-72.25, 64.2)
  line L1 (-72.25, 64.2) -> (-77.45, 64.2)
  line L2 (-77.45, 64.2) -> (-77.45, 60)
  line L3 (-77.45, 60) -> (-72.25, 60)
  line L4 (-59.55, 60) -> (-59.55, 64.2)
  line L5 (-59.55, 64.2) -> (-64.75, 64.2)
  line L6 (-64.75, 64.2) -> (-64.75, 60)
  line L7 (-64.75, 60) -> (-59.55, 60)
extrude "ToF posts SRL" add sketch "ToF posts SRL sketch" along normal blind 5.2 from surface at 110.36 bodies 44 in component "Upper frame"
sketch "ToF pilots SRL sketch" plane through (0, 0, 0) normal (0, 0, 1) x (1, 0, 0) in component "Upper frame"
  line L0 (-73.75, 59.5) -> (-73.75, 64.5)
  line L1 (-73.75, 64.5) -> (-75.95, 64.5)
  line L2 (-75.95, 64.5) -> (-75.95, 59.5)
  line L3 (-75.95, 59.5) -> (-73.75, 59.5)
  line L4 (-61.05, 59.5) -> (-61.05, 64.5)
  line L5 (-61.05, 64.5) -> (-63.25, 64.5)
  line L6 (-63.25, 64.5) -> (-63.25, 59.5)
  line L7 (-63.25, 59.5) -> (-61.05, 59.5)
extrude "ToF pilots SRL" cut sketch "ToF pilots SRL sketch" along normal blind 2.2 from surface at 111.86 bodies 44 in component "Upper frame"
sketch "ToF screw access SRL sketch" plane through (0, 0, 0) normal (0, 0, 1) x (1, 0, 0) in component "Upper frame"
  line L0 (-72.35, 52.6) -> (-72.35, 56.3)
  line L1 (-72.35, 56.3) -> (-77.35, 56.3)
  line L2 (-77.35, 56.3) -> (-77.35, 52.6)
  line L3 (-77.35, 52.6) -> (-72.35, 52.6)
  line L4 (-59.65, 52.6) -> (-59.65, 56.3)
  line L5 (-59.65, 56.3) -> (-64.65, 56.3)
  line L6 (-64.65, 56.3) -> (-64.65, 52.6)
  line L7 (-64.65, 52.6) -> (-59.65, 52.6)
extrude "ToF screw access SRL" cut sketch "ToF screw access SRL sketch" along normal blind 5 from surface at 110.46 bodies 44 in component "Upper frame"
sketch "ToF pocket SRR sketch" plane through (0, 0, 0) normal (0, 0, 1) x (1, 0, 0) in component "Upper frame"
  line L0 (-78.19, -56.1) -> (-78.19, -63.6)
  line L1 (-78.19, -63.6) -> (-58.81, -63.6)
  line L2 (-58.81, -63.6) -> (-58.81, -56.1)
  line L3 (-58.81, -56.1) -> (-78.19, -56.1)
extrude "ToF pocket SRR" cut sketch "ToF pocket SRR sketch" along normal blind 28 from surface at 90 bodies 44 in component "Upper frame"
sketch "ToF plug shaft SRR sketch" plane through (0, 0, 0) normal (0, 0, 1) x (1, 0, 0) in component "Upper frame"
  line L0 (-72.3, -59.5) -> (-72.3, -64)
  line L1 (-72.3, -64) -> (-64.7, -64)
  line L2 (-64.7, -64) -> (-64.7, -59.5)
  line L3 (-64.7, -59.5) -> (-72.3, -59.5)
extrude "ToF plug shaft SRR" cut sketch "ToF plug shaft SRR sketch" along normal blind 4.5 from surface at 86 bodies 44 in component "Upper frame"
sketch "ToF tunnel SRR sketch" plane through (0, 0, 0) normal (0, 0, 1) x (1, 0, 0) in component "Upper frame"
  line L0 (-77.5, -63.1) -> (-77.5, -100)
  line L1 (-77.5, -100) -> (-59.5, -100)
  line L2 (-59.5, -100) -> (-59.5, -63.1)
  line L3 (-59.5, -63.1) -> (-77.5, -63.1)
extrude "ToF tunnel SRR" cut sketch "ToF tunnel SRR sketch" along normal blind 18 from surface at 93.8 bodies 44 in component "Upper frame"
sketch "ToF posts SRR sketch" plane through (0, 0, 0) normal (0, 0, 1) x (1, 0, 0) in component "Upper frame"
  line L0 (-64.75, -60) -> (-64.75, -64.2)
  line L1 (-64.75, -64.2) -> (-59.55, -64.2)
  line L2 (-59.55, -64.2) -> (-59.55, -60)
  line L3 (-59.55, -60) -> (-64.75, -60)
  line L4 (-77.45, -60) -> (-77.45, -64.2)
  line L5 (-77.45, -64.2) -> (-72.25, -64.2)
  line L6 (-72.25, -64.2) -> (-72.25, -60)
  line L7 (-72.25, -60) -> (-77.45, -60)
extrude "ToF posts SRR" add sketch "ToF posts SRR sketch" along normal blind 5.2 from surface at 110.36 bodies 44 in component "Upper frame"
sketch "ToF pilots SRR sketch" plane through (0, 0, 0) normal (0, 0, 1) x (1, 0, 0) in component "Upper frame"
  line L0 (-63.25, -59.5) -> (-63.25, -64.5)
  line L1 (-63.25, -64.5) -> (-61.05, -64.5)
  line L2 (-61.05, -64.5) -> (-61.05, -59.5)
  line L3 (-61.05, -59.5) -> (-63.25, -59.5)
  line L4 (-75.95, -59.5) -> (-75.95, -64.5)
  line L5 (-75.95, -64.5) -> (-73.75, -64.5)
  line L6 (-73.75, -64.5) -> (-73.75, -59.5)
  line L7 (-73.75, -59.5) -> (-75.95, -59.5)
extrude "ToF pilots SRR" cut sketch "ToF pilots SRR sketch" along normal blind 2.2 from surface at 111.86 bodies 44 in component "Upper frame"
sketch "ToF screw access SRR sketch" plane through (0, 0, 0) normal (0, 0, 1) x (1, 0, 0) in component "Upper frame"
  line L0 (-64.65, -52.6) -> (-64.65, -56.3)
  line L1 (-64.65, -56.3) -> (-59.65, -56.3)
  line L2 (-59.65, -56.3) -> (-59.65, -52.6)
  line L3 (-59.65, -52.6) -> (-64.65, -52.6)
  line L4 (-77.35, -52.6) -> (-77.35, -56.3)
  line L5 (-77.35, -56.3) -> (-72.35, -56.3)
  line L6 (-72.35, -56.3) -> (-72.35, -52.6)
  line L7 (-72.35, -52.6) -> (-77.35, -52.6)
extrude "ToF screw access SRR" cut sketch "ToF screw access SRR sketch" along normal blind 5 from surface at 110.46 bodies 44 in component "Upper frame"
sketch "ToF pocket RL sketch" plane through (0, 0, 0) normal (0, 0, 1) x (1, 0, 0) in component "Upper frame"
  line L0 (-80.1, 45.69) -> (-87.6, 45.69)
  line L1 (-87.6, 45.69) -> (-87.6, 26.31)
  line L2 (-87.6, 26.31) -> (-80.1, 26.31)
  line L3 (-80.1, 26.31) -> (-80.1, 45.69)
extrude "ToF pocket RL" cut sketch "ToF pocket RL sketch" along normal blind 28 from surface at 90 bodies 44 in component "Upper frame"
sketch "ToF plug shaft RL sketch" plane through (0, 0, 0) normal (0, 0, 1) x (1, 0, 0) in component "Upper frame"
  line L0 (-83.5, 39.8) -> (-88, 39.8)
  line L1 (-88, 39.8) -> (-88, 32.2)
  line L2 (-88, 32.2) -> (-83.5, 32.2)
  line L3 (-83.5, 32.2) -> (-83.5, 39.8)
extrude "ToF plug shaft RL" cut sketch "ToF plug shaft RL sketch" along normal blind 4.5 from surface at 86 bodies 44 in component "Upper frame"
sketch "ToF tunnel RL sketch" plane through (0, 0, 0) normal (0, 0, 1) x (1, 0, 0) in component "Upper frame"
  line L0 (-87.1, 45) -> (-124, 45)
  line L1 (-124, 45) -> (-124, 27)
  line L2 (-124, 27) -> (-87.1, 27)
  line L3 (-87.1, 27) -> (-87.1, 45)
extrude "ToF tunnel RL" cut sketch "ToF tunnel RL sketch" along normal blind 18 from surface at 93.8 bodies 44 in component "Upper frame"
sketch "ToF posts RL sketch" plane through (0, 0, 0) normal (0, 0, 1) x (1, 0, 0) in component "Upper frame"
  line L0 (-84, 32.25) -> (-88.2, 32.25)
  line L1 (-88.2, 32.25) -> (-88.2, 27.05)
  line L2 (-88.2, 27.05) -> (-84, 27.05)
  line L3 (-84, 27.05) -> (-84, 32.25)
  line L4 (-84, 44.95) -> (-88.2, 44.95)
  line L5 (-88.2, 44.95) -> (-88.2, 39.75)
  line L6 (-88.2, 39.75) -> (-84, 39.75)
  line L7 (-84, 39.75) -> (-84, 44.95)
extrude "ToF posts RL" add sketch "ToF posts RL sketch" along normal blind 5.2 from surface at 110.36 bodies 44 in component "Upper frame"
sketch "ToF pilots RL sketch" plane through (0, 0, 0) normal (0, 0, 1) x (1, 0, 0) in component "Upper frame"
  line L0 (-83.5, 30.75) -> (-88.5, 30.75)
  line L1 (-88.5, 30.75) -> (-88.5, 28.55)
  line L2 (-88.5, 28.55) -> (-83.5, 28.55)
  line L3 (-83.5, 28.55) -> (-83.5, 30.75)
  line L4 (-83.5, 43.45) -> (-88.5, 43.45)
  line L5 (-88.5, 43.45) -> (-88.5, 41.25)
  line L6 (-88.5, 41.25) -> (-83.5, 41.25)
  line L7 (-83.5, 41.25) -> (-83.5, 43.45)
extrude "ToF pilots RL" cut sketch "ToF pilots RL sketch" along normal blind 2.2 from surface at 111.86 bodies 44 in component "Upper frame"
sketch "ToF screw access RL sketch" plane through (0, 0, 0) normal (0, 0, 1) x (1, 0, 0) in component "Upper frame"
  line L0 (-76.6, 32.15) -> (-80.3, 32.15)
  line L1 (-80.3, 32.15) -> (-80.3, 27.15)
  line L2 (-80.3, 27.15) -> (-76.6, 27.15)
  line L3 (-76.6, 27.15) -> (-76.6, 32.15)
  line L4 (-76.6, 44.85) -> (-80.3, 44.85)
  line L5 (-80.3, 44.85) -> (-80.3, 39.85)
  line L6 (-80.3, 39.85) -> (-76.6, 39.85)
  line L7 (-76.6, 39.85) -> (-76.6, 44.85)
extrude "ToF screw access RL" cut sketch "ToF screw access RL sketch" along normal blind 5 from surface at 110.46 bodies 44 in component "Upper frame"
sketch "ToF pocket RR sketch" plane through (0, 0, 0) normal (0, 0, 1) x (1, 0, 0) in component "Upper frame"
  line L0 (-80.1, -26.31) -> (-87.6, -26.31)
  line L1 (-87.6, -26.31) -> (-87.6, -45.69)
  line L2 (-87.6, -45.69) -> (-80.1, -45.69)
  line L3 (-80.1, -45.69) -> (-80.1, -26.31)
extrude "ToF pocket RR" cut sketch "ToF pocket RR sketch" along normal blind 28 from surface at 90 bodies 44 in component "Upper frame"
sketch "ToF plug shaft RR sketch" plane through (0, 0, 0) normal (0, 0, 1) x (1, 0, 0) in component "Upper frame"
  line L0 (-83.5, -32.2) -> (-88, -32.2)
  line L1 (-88, -32.2) -> (-88, -39.8)
  line L2 (-88, -39.8) -> (-83.5, -39.8)
  line L3 (-83.5, -39.8) -> (-83.5, -32.2)
extrude "ToF plug shaft RR" cut sketch "ToF plug shaft RR sketch" along normal blind 4.5 from surface at 86 bodies 44 in component "Upper frame"
sketch "ToF tunnel RR sketch" plane through (0, 0, 0) normal (0, 0, 1) x (1, 0, 0) in component "Upper frame"
  line L0 (-87.1, -27) -> (-124, -27)
  line L1 (-124, -27) -> (-124, -45)
  line L2 (-124, -45) -> (-87.1, -45)
  line L3 (-87.1, -45) -> (-87.1, -27)
extrude "ToF tunnel RR" cut sketch "ToF tunnel RR sketch" along normal blind 18 from surface at 93.8 bodies 44 in component "Upper frame"
sketch "ToF posts RR sketch" plane through (0, 0, 0) normal (0, 0, 1) x (1, 0, 0) in component "Upper frame"
  line L0 (-84, -39.75) -> (-88.2, -39.75)
  line L1 (-88.2, -39.75) -> (-88.2, -44.95)
  line L2 (-88.2, -44.95) -> (-84, -44.95)
  line L3 (-84, -44.95) -> (-84, -39.75)
  line L4 (-84, -27.05) -> (-88.2, -27.05)
  line L5 (-88.2, -27.05) -> (-88.2, -32.25)
  line L6 (-88.2, -32.25) -> (-84, -32.25)
  line L7 (-84, -32.25) -> (-84, -27.05)
extrude "ToF posts RR" add sketch "ToF posts RR sketch" along normal blind 5.2 from surface at 110.36 bodies 44 in component "Upper frame"
sketch "ToF pilots RR sketch" plane through (0, 0, 0) normal (0, 0, 1) x (1, 0, 0) in component "Upper frame"
  line L0 (-83.5, -41.25) -> (-88.5, -41.25)
  line L1 (-88.5, -41.25) -> (-88.5, -43.45)
  line L2 (-88.5, -43.45) -> (-83.5, -43.45)
  line L3 (-83.5, -43.45) -> (-83.5, -41.25)
  line L4 (-83.5, -28.55) -> (-88.5, -28.55)
  line L5 (-88.5, -28.55) -> (-88.5, -30.75)
  line L6 (-88.5, -30.75) -> (-83.5, -30.75)
  line L7 (-83.5, -30.75) -> (-83.5, -28.55)
extrude "ToF pilots RR" cut sketch "ToF pilots RR sketch" along normal blind 2.2 from surface at 111.86 bodies 44 in component "Upper frame"
sketch "ToF screw access RR sketch" plane through (0, 0, 0) normal (0, 0, 1) x (1, 0, 0) in component "Upper frame"
  line L0 (-76.6, -39.85) -> (-80.3, -39.85)
  line L1 (-80.3, -39.85) -> (-80.3, -44.85)
  line L2 (-80.3, -44.85) -> (-76.6, -44.85)
  line L3 (-76.6, -44.85) -> (-76.6, -39.85)
  line L4 (-76.6, -27.15) -> (-80.3, -27.15)
  line L5 (-80.3, -27.15) -> (-80.3, -32.15)
  line L6 (-80.3, -32.15) -> (-76.6, -32.15)
  line L7 (-76.6, -32.15) -> (-76.6, -27.15)
extrude "ToF screw access RR" cut sketch "ToF screw access RR sketch" along normal blind 5 from surface at 110.46 bodies 44 in component "Upper frame"
sketch "Camera window L sketch" plane through (0, 0, 0) normal (0, 1, 0) x (1, 0, 0) in component "Upper frame"
  line L0 (-10.9288, -86) -> (17.0712, -86)
  line L1 (17.0712, -86) -> (17.0712, -106)
  line L2 (17.0712, -106) -> (-10.9288, -106)
  line L3 (-10.9288, -106) -> (-10.9288, -86)
extrude "Camera window L" cut sketch "Camera window L sketch" along normal blind 24 from surface at 84 bodies 44 in component "Upper frame"
sketch "Camera window R sketch" plane through (0, 0, 0) normal (0, 1, 0) x (1, 0, 0) in component "Upper frame"
  line L0 (-10.9288, -86) -> (17.0712, -86)
  line L1 (17.0712, -86) -> (17.0712, -106)
  line L2 (17.0712, -106) -> (-10.9288, -106)
  line L3 (-10.9288, -106) -> (-10.9288, -86)
extrude "Camera window R" cut sketch "Camera window R sketch" along normal blind 24 from surface at -108 bodies 44 in component "Upper frame"
sketch "Camera insert holes L sketch" plane through (0, 0, 0) normal (0, 0, 1) x (1, 0, 0) in component "Upper frame"
  line L0 (26.0712, 84.5103) -> (30.0712, 84.5103)
  line L1 (30.0712, 84.5103) -> (30.0712, 91.5103)
  line L2 (30.0712, 91.5103) -> (26.0712, 91.5103)
  line L3 (26.0712, 91.5103) -> (26.0712, 84.5103)
  line L4 (-23.9288, 86.2876) -> (-19.9288, 86.2876)
  line L5 (-19.9288, 86.2876) -> (-19.9288, 93.2876)
  line L6 (-19.9288, 93.2876) -> (-23.9288, 93.2876)
  line L7 (-23.9288, 93.2876) -> (-23.9288, 86.2876)
extrude "Camera insert holes L" cut sketch "Camera insert holes L sketch" along normal blind 4 from surface at 93 bodies 44 in component "Upper frame"
sketch "Camera insert holes R sketch" plane through (0, 0, 0) normal (0, 0, 1) x (1, 0, 0) in component "Upper frame"
  line L0 (26.0712, -91.5103) -> (30.0712, -91.5103)
  line L1 (30.0712, -91.5103) -> (30.0712, -84.5103)
  line L2 (30.0712, -84.5103) -> (26.0712, -84.5103)
  line L3 (26.0712, -84.5103) -> (26.0712, -91.5103)
  line L4 (-23.9288, -93.2876) -> (-19.9288, -93.2876)
  line L5 (-19.9288, -93.2876) -> (-19.9288, -86.2876)
  line L6 (-19.9288, -86.2876) -> (-23.9288, -86.2876)
  line L7 (-23.9288, -86.2876) -> (-23.9288, -93.2876)
extrude "Camera insert holes R" cut sketch "Camera insert holes R sketch" along normal blind 4 from surface at 93 bodies 44 in component "Upper frame"
sketch "VL53L0X board F sketch" plane through (0, 0, 0) normal (0, 0, 1) x (1, 0, 0) in component "ToF F"
  line L0 (93.4, -8.89) -> (95, -8.89)
  line L1 (95, -8.89) -> (95, 8.89)
  line L2 (95, 8.89) -> (93.4, 8.89)
  line L3 (93.4, 8.89) -> (93.4, -8.89)
extrude "VL53L0X board F" add sketch "VL53L0X board F sketch" along normal blind 25.4 from surface at 90.1 separate body makes body 45 in component "ToF F"
sketch "Board holes sketch" plane through (0, 0, 0) normal (0, 0, 1) x (1, 0, 0) in component "ToF F"
  line L0 (92.9, 5.1) -> (95.5, 5.1)
  line L1 (95.5, 5.1) -> (95.5, 7.6)
  line L2 (95.5, 7.6) -> (92.9, 7.6)
  line L3 (92.9, 7.6) -> (92.9, 5.1)
  line L4 (92.9, -7.6) -> (95.5, -7.6)
  line L5 (95.5, -7.6) -> (95.5, -5.1)
  line L6 (95.5, -5.1) -> (92.9, -5.1)
  line L7 (92.9, -5.1) -> (92.9, -7.6)
extrude "Board holes" cut sketch "Board holes sketch" along normal blind 2.5 from surface at 111.71 bodies 45 in component "ToF F"
sketch "Board holes sketch (1)" plane through (0, 0, 0) normal (0, 0, 1) x (1, 0, 0) in component "ToF F"
  line L0 (92.9, 5.1) -> (95.5, 5.1)
  line L1 (95.5, 5.1) -> (95.5, 7.6)
  line L2 (95.5, 7.6) -> (92.9, 7.6)
  line L3 (92.9, 7.6) -> (92.9, 5.1)
  line L4 (92.9, -7.6) -> (95.5, -7.6)
  line L5 (95.5, -7.6) -> (95.5, -5.1)
  line L6 (95.5, -5.1) -> (92.9, -5.1)
  line L7 (92.9, -5.1) -> (92.9, -7.6)
extrude "Board holes (1)" cut sketch "Board holes sketch (1)" along normal blind 2.5 from surface at 91.39 bodies 45 in component "ToF F"
sketch "QT connector F sketch" plane through (0, 0, 0) normal (0, 0, 1) x (1, 0, 0) in component "ToF F"
  line L0 (95, -3.05) -> (98.05, -3.05)
  line L1 (98.05, -3.05) -> (98.05, 3.05)
  line L2 (98.05, 3.05) -> (95, 3.05)
  line L3 (95, 3.05) -> (95, -3.05)
extrude "QT connector F" add sketch "QT connector F sketch" along normal blind 4.25 from surface at 110.67 separate body makes body 46 in component "ToF F"
sketch "QT connector F sketch (1)" plane through (0, 0, 0) normal (0, 0, 1) x (1, 0, 0) in component "ToF F"
  line L0 (95, -3.05) -> (98.05, -3.05)
  line L1 (98.05, -3.05) -> (98.05, 3.05)
  line L2 (98.05, 3.05) -> (95, 3.05)
  line L3 (95, 3.05) -> (95, -3.05)
extrude "QT connector F (1)" add sketch "QT connector F sketch (1)" along normal blind 4.25 from surface at 90.68 separate body makes body 47 in component "ToF F"
sketch "VL53L0X chip F sketch" plane through (0, 0, 0) normal (0, 0, 1) x (1, 0, 0) in component "ToF F"
  line L0 (95, -2.2) -> (96, -2.2)
  line L1 (96, -2.2) -> (96, 2.2)
  line L2 (96, 2.2) -> (95, 2.2)
  line L3 (95, 2.2) -> (95, -2.2)
extrude "VL53L0X chip F" add sketch "VL53L0X chip F sketch" along normal blind 2.4 from surface at 101.6 separate body makes body 48 in component "ToF F"
sketch "M2.5 screw heads F sketch" plane through (0, 0, 0) normal (0, 0, 1) x (1, 0, 0) in component "ToF F"
  line L0 (91.9, 4.1) -> (93.4, 4.1)
  line L1 (93.4, 4.1) -> (93.4, 8.6)
  line L2 (93.4, 8.6) -> (91.9, 8.6)
  line L3 (91.9, 8.6) -> (91.9, 4.1)
  line L4 (91.9, -8.6) -> (93.4, -8.6)
  line L5 (93.4, -8.6) -> (93.4, -4.1)
  line L6 (93.4, -4.1) -> (91.9, -4.1)
  line L7 (91.9, -4.1) -> (91.9, -8.6)
extrude "M2.5 screw heads F" add sketch "M2.5 screw heads F sketch" along normal blind 4.5 from surface at 110.71 separate body makes body 49 at (93.4, 5.6, 112.21) makes body 50 at (93.4, -7.1, 112.21) in component "ToF F"
sketch "M2.5 screw shafts F sketch" plane through (0, 0, 0) normal (0, 0, 1) x (1, 0, 0) in component "ToF F"
  line L0 (93.4, 5.35) -> (99.4, 5.35)
  line L1 (99.4, 5.35) -> (99.4, 7.35)
  line L2 (99.4, 7.35) -> (93.4, 7.35)
  line L3 (93.4, 7.35) -> (93.4, 5.35)
  line L4 (93.4, -7.35) -> (99.4, -7.35)
  line L5 (99.4, -7.35) -> (99.4, -5.35)
  line L6 (99.4, -5.35) -> (93.4, -5.35)
  line L7 (93.4, -5.35) -> (93.4, -7.35)
extrude "M2.5 screw shafts F" add sketch "M2.5 screw shafts F sketch" along normal blind 2 from surface at 111.96 separate body makes body 51 at (97.4, 7.35, 112.6267) makes body 52 at (97.4, -5.35, 112.6267) in component "ToF F"
sketch "VL53L0X board FL sketch" plane through (0, 0, 0) normal (0, 0, 1) x (1, 0, 0) in component "ToF FL"
  line L0 (91.8344, 31.1269) -> (93.2845, 31.8031)
  line L1 (93.2845, 31.8031) -> (85.7704, 47.9173)
  line L2 (85.7704, 47.9173) -> (84.3203, 47.2411)
  line L3 (84.3203, 47.2411) -> (91.8344, 31.1269)
extrude "VL53L0X board FL" add sketch "VL53L0X board FL sketch" along normal blind 25.4 from surface at 90.1 separate body makes body 53 in component "ToF FL"
sketch "Board holes sketch (2)" plane through (0, 0, 0) normal (0, 0, 1) x (1, 0, 0) in component "ToF FL"
  line L0 (85.4689, 43.5949) -> (87.8253, 44.6937)
  line L1 (87.8253, 44.6937) -> (86.7687, 46.9594)
  line L2 (86.7687, 46.9594) -> (84.4123, 45.8606)
  line L3 (84.4123, 45.8606) -> (85.4689, 43.5949)
  line L4 (90.8361, 32.0848) -> (93.1925, 33.1836)
  line L5 (93.1925, 33.1836) -> (92.136, 35.4493)
  line L6 (92.136, 35.4493) -> (89.7796, 34.3505)
  line L7 (89.7796, 34.3505) -> (90.8361, 32.0848)
extrude "Board holes'" cut sketch "Board holes sketch (2)" along normal blind 2.5 from surface at 111.71 bodies 53 in component "ToF FL"
sketch "Board holes sketch (1) (2)" plane through (0, 0, 0) normal (0, 0, 1) x (1, 0, 0) in component "ToF FL"
  line L0 (85.4689, 43.5949) -> (87.8253, 44.6937)
  line L1 (87.8253, 44.6937) -> (86.7687, 46.9594)
  line L2 (86.7687, 46.9594) -> (84.4123, 45.8606)
  line L3 (84.4123, 45.8606) -> (85.4689, 43.5949)
  line L4 (90.8361, 32.0848) -> (93.1925, 33.1836)
  line L5 (93.1925, 33.1836) -> (92.136, 35.4493)
  line L6 (92.136, 35.4493) -> (89.7796, 34.3505)
  line L7 (89.7796, 34.3505) -> (90.8361, 32.0848)
extrude "Board holes (1)'" cut sketch "Board holes sketch (1) (2)" along normal blind 2.5 from surface at 91.39 bodies 53 in component "ToF FL"
sketch "QT connector FL sketch" plane through (0, 0, 0) normal (0, 0, 1) x (1, 0, 0) in component "ToF FL"
  line L0 (90.8164, 37.096) -> (93.5807, 38.3849)
  line L1 (93.5807, 38.3849) -> (91.0027, 43.9134)
  line L2 (91.0027, 43.9134) -> (88.2385, 42.6244)
  line L3 (88.2385, 42.6244) -> (90.8164, 37.096)
extrude "QT connector FL" add sketch "QT connector FL sketch" along normal blind 4.25 from surface at 110.67 separate body makes body 54 in component "ToF FL"
sketch "QT connector FL sketch (1)" plane through (0, 0, 0) normal (0, 0, 1) x (1, 0, 0) in component "ToF FL"
  line L0 (90.8164, 37.096) -> (93.5807, 38.3849)
  line L1 (93.5807, 38.3849) -> (91.0027, 43.9134)
  line L2 (91.0027, 43.9134) -> (88.2385, 42.6244)
  line L3 (88.2385, 42.6244) -> (90.8164, 37.096)
extrude "QT connector FL (1)" add sketch "QT connector FL sketch (1)" along normal blind 4.25 from surface at 90.68 separate body makes body 55 in component "ToF FL"
sketch "VL53L0X chip FL sketch" plane through (0, 0, 0) normal (0, 0, 1) x (1, 0, 0) in component "ToF FL"
  line L0 (90.4572, 37.8663) -> (91.3635, 38.2889)
  line L1 (91.3635, 38.2889) -> (89.504, 42.2767)
  line L2 (89.504, 42.2767) -> (88.5977, 41.8541)
  line L3 (88.5977, 41.8541) -> (90.4572, 37.8663)